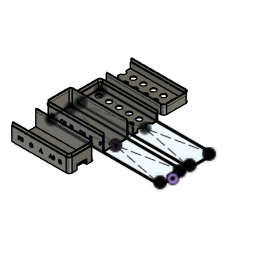
harpcase_v3 (Autodesk Fusion 360 design; units mm, degrees)
Autodesk Fusion 360 part; units mm, degrees
sketch "Sketch1" plane through (0, 0, 0) normal (0, 0, 1) x (1, 0, 0)
  line L0 (167.5, 35) -> (-167.5, 35)
  line L1 (-172.5, 30) -> (-172.5, -30)
  line L2 (-167.5, -35) -> (167.5, -35)
  line L3 (172.5, -30) -> (172.5, 30)
  line L4 (172.5, 35) -> (-172.5, -35) construction
  line L5 (-172.5, 35) -> (172.5, -35) construction
  line L6 (0, 0) -> (0, 91) construction
  line L7 (167.5, 126) -> (-167.5, 126)
  line L8 (-172.5, 121) -> (-172.5, 61)
  line L9 (-167.5, 56) -> (167.5, 56)
  line L10 (172.5, 61) -> (172.5, 121)
  line L11 (172.5, 126) -> (-172.5, 56) construction
  line L12 (-172.5, 126) -> (172.5, 56) construction
  arc A0 (-167.5, 126) -> (-172.5, 121) centre (-167.5, 121) ccw
  arc A1 (172.5, 121) -> (167.5, 126) centre (167.5, 121) ccw
  arc A2 (167.5, 56) -> (172.5, 61) centre (167.5, 61) ccw
  arc A3 (-172.5, 61) -> (-167.5, 56) centre (-167.5, 61) ccw
  arc A4 (-167.5, 35) -> (-172.5, 30) centre (-167.5, 30) ccw
  arc A5 (-172.5, -30) -> (-167.5, -35) centre (-167.5, -30) ccw
  arc A6 (167.5, -35) -> (172.5, -30) centre (167.5, -30) ccw
  arc A7 (172.5, 30) -> (167.5, 35) centre (167.5, 30) ccw
  line L13 (-176.5417, 121) -> (-176.5417, 61)
  arc A8 (-176.5417, 61) -> (-167.5, 51.9583) centre (-167.5, 61) ccw
  line L14 (-167.5, 51.9583) -> (167.5, 51.9583)
  arc A9 (167.5, 51.9583) -> (176.5417, 61) centre (167.5, 61) ccw
  line L15 (176.5417, 61) -> (176.5417, 121)
  arc A10 (176.5417, 121) -> (167.5, 130.0417) centre (167.5, 121) ccw
  line L16 (167.5, 130.0417) -> (-167.5, 130.0417)
  arc A11 (-167.5, 130.0417) -> (-176.5417, 121) centre (-167.5, 121) ccw
  line L17 (-174.5208, 121) -> (-174.5208, 61)
  arc A12 (-174.5208, 61) -> (-167.5, 53.9792) centre (-167.5, 61) ccw
  line L18 (-167.5, 53.9792) -> (167.5, 53.9792)
  arc A13 (167.5, 53.9792) -> (174.5208, 61) centre (167.5, 61) ccw
  line L19 (174.5208, 61) -> (174.5208, 121)
  arc A14 (174.5208, 121) -> (167.5, 128.0208) centre (167.5, 121) ccw
  line L20 (167.5, 128.0208) -> (-167.5, 128.0208)
  arc A15 (-167.5, 128.0208) -> (-174.5208, 121) centre (-167.5, 121) ccw
  line L21 (-176.5417, 30) -> (-176.5417, -30)
  arc A16 (-176.5417, -30) -> (-167.5, -39.0417) centre (-167.5, -30) ccw
  line L22 (-167.5, -39.0417) -> (167.5, -39.0417)
  arc A17 (167.5, -39.0417) -> (176.5417, -30) centre (167.5, -30) ccw
  line L23 (176.5417, -30) -> (176.5417, 30)
  arc A18 (176.5417, 30) -> (167.5, 39.0417) centre (167.5, 30) ccw
  line L24 (167.5, 39.0417) -> (-167.5, 39.0417)
  arc A19 (-167.5, 39.0417) -> (-176.5417, 30) centre (-167.5, 30) ccw
  line L25 (-174.5208, 30) -> (-174.5208, -30)
  arc A20 (-174.5208, -30) -> (-167.5, -37.0208) centre (-167.5, -30) ccw
  line L26 (-167.5, -37.0208) -> (167.5, -37.0208)
  arc A21 (167.5, -37.0208) -> (174.5208, -30) centre (167.5, -30) ccw
  line L27 (174.5208, -30) -> (174.5208, 30)
  arc A22 (174.5208, 30) -> (167.5, 37.0208) centre (167.5, 30) ccw
  line L28 (167.5, 37.0208) -> (-167.5, 37.0208)
  arc A23 (-167.5, 37.0208) -> (-174.5208, 30) centre (-167.5, 30) ccw
  point P0 (0, 91)
  dimension "d5" = 345
  dimension "d6" = 70
  dimension "d7" = 91
  dimension "d8" = 345
  dimension "d9" = 70
  dimension "d11" = 5
  dimension "d12" = 5
  dimension "d14" = 4.0417
  dimension "d15" = 2.0208
  dimension "d16" = 4.0417
  dimension "d17" = 2.0208
  constraint horizontal L0
  constraint perpendicular L0 L1
  constraint parallel L0 L2
  constraint parallel L1 L3
  constraint coincident L4 L6.start
  constraint coincident L5 L6.start
  constraint coincident L6.start origin
  constraint perpendicular L0 L6
  constraint horizontal L7
  constraint perpendicular L7 L8
  constraint parallel L7 L9
  constraint parallel L8 L10
  constraint coincident L11 P0
  constraint coincident L12 P0
  constraint coincident P0 L6.end
  constraint coincident L12.start L8
  constraint coincident L12.start L7
  constraint tangent L8 A0
  constraint tangent L7 A0
  constraint coincident L11.start L7
  constraint coincident L11.start L10
  constraint tangent L7 A1
  constraint tangent L10 A1
  constraint equal A0 A1
  constraint coincident L12.end L9
  constraint coincident L12.end L10
  constraint tangent L9 A2
  constraint tangent L10 A2
  constraint equal A0 A2
  constraint coincident L11.end L9
  constraint coincident L11.end L8
  constraint tangent L9 A3
  constraint tangent L8 A3
  constraint equal A0 A3
  constraint coincident L5.start L1
  constraint coincident L5.start L0
  constraint tangent L1 A4
  constraint tangent L0 A4
  constraint coincident L4.end L2
  constraint coincident L4.end L1
  constraint tangent L2 A5
  constraint tangent L1 A5
  constraint equal A4 A5
  constraint coincident L5.end L2
  constraint coincident L5.end L3
  constraint tangent L2 A6
  constraint tangent L3 A6
  constraint equal A4 A6
  constraint coincident L4.start L0
  constraint coincident L4.start L3
  constraint tangent L0 A7
  constraint tangent L3 A7
  constraint equal A4 A7
  measures "d5" distance of L4.end L5.end
  measures "d6" distance of L5.start L4.end
  measures "d7" distance of L6.start P0
  measures "d8" distance of L11.end L12.end
  measures "d9" distance of L12.start L11.end
  measures "d11" radius of A0
  measures "d12" radius of A4
extrude "Extrude1" add sketch "Sketch1" along normal blind 2.425 contours L0 L1 L2 L3 A4 A5 A6 A7 | L7 L8 L9 L10 A0 A1 A2 A3 makes body 1 at (55.8333, 79.3333, 0) makes body 2 at (55.8333, -11.6667, 0)
extrude "Extrude2" add sketch "Sketch1" along normal blind 50.4 contours L25 A20 L26 A21 L27 A22 L28 A23 bodies 2
extrude "Extrude3" add sketch "Sketch1" along normal blind 42 contours L21 A16 L22 A17 L23 A18 L24 A19 bodies 2
extrude "Extrude4" add sketch "Sketch1" along normal blind 19.6 contours L17 A12 L18 A13 L19 A14 L20 A15 bodies 1
extrude "Extrude5" add sketch "Sketch1" along normal blind 28 contours L13 A8 L14 A9 L15 A10 L16 A11 bodies 1
ref_plane "WorkPlane1" through (176.5417, 0, 21) normal (1, 0, 0) x (0, 1, 0)
sketch "Sketch2" plane through (176.5417, 0, 0) normal (1, 0, 0) x (0, 1, 0)
  line L0 (0, 0) -> (15, 0)
  line L1 (15, 0) -> (15, 15)
  line L2 (15, 15) -> (0, 15)
  line L3 (0, 15) -> (0, 0)
  line L4 (0, 0) -> (-15, 0)
  line L5 (-15, 0) -> (-15, 15)
  line L6 (-15, 15) -> (0, 15)
  line L7 (0, 15) -> (0, 0)
  dimension "d35" = 15
  dimension "d36" = 15
  dimension "d38" = 15
  dimension "d39" = 15
  constraint horizontal L0
  constraint vertical L1
  constraint horizontal L2
  constraint vertical L3
  constraint coincident L0.start L3.end
  constraint horizontal L4
  constraint vertical L5
  constraint horizontal L6
  constraint vertical L7
  measures "d35" distance of L0.start L0.end
  measures "d36" distance of L0.start L2.end
  measures "d38" distance of L0.start L4.end
  measures "d39" distance of L0.start L2.end
extrude "Extrude6" cut sketch "Sketch2" against normal blind 10 bodies 2
ref_plane "WorkPlane2" through (0, 91, 2.425) normal (0, 0, 1) x (1, 0, 0)
sketch "Sketch3" plane through (0, 0, 2.425) normal (0, 0, 1) x (1, 0, 0)
  line L0 (167.5, 126) -> (-167.5, 126)
  line L1 (-172.5, 121) -> (-172.5, 61)
  line L2 (-167.5, 56) -> (172.5, 56)
  line L3 (172.5, 62.1164) -> (172.5, 121)
  line L4 (172.5, 126) -> (-172.5, 56) construction
  line L5 (-172.5, 126) -> (166.5058, 57.2162) construction
  arc A0 (-167.5, 126) -> (-172.5, 121) centre (-167.5, 121) ccw
  arc A1 (-172.5, 61) -> (-167.5, 56) centre (-167.5, 61) ccw
  arc A2 (166.5058, 57.2162) -> (172.5, 62.1164) centre (167.5, 62.1164) ccw
  arc A3 (172.5, 121) -> (167.5, 126) centre (167.5, 121) ccw
  line L6 (0, 126) -> (0, 56) construction
  line L7 (172.5, 91.5582) -> (-172.5, 91) construction
  line L8 (0, 56) -> (-155, 56) construction
  line L9 (-172.5, 91) -> (-172.4741, 75) construction
  line L10 (-155, 56) -> (-155, 77.7) construction
  circle A4 centre (-155, 77.7) radius 8.1
  line L11 (-155, 77.7) -> (-155.043, 104.3) construction
  circle A5 centre (-155.043, 104.3) radius 8.1
  circle A6 centre (-124.043, 104.3) radius 8.1
  circle A7 centre (-124, 77.7) radius 8.1
  circle A8 centre (-93.043, 104.3) radius 8.1
  circle A9 centre (-93, 77.7) radius 8.1
  circle A10 centre (-62.043, 104.3) radius 8.1
  circle A11 centre (-62, 77.7) radius 8.1
  circle A12 centre (-31.043, 104.3) radius 8.1
  circle A13 centre (-31, 77.7) radius 8.1
  circle A14 centre (-0.043, 104.3) radius 8.1
  circle A15 centre (0, 77.7) radius 8.1
  circle A16 centre (30.957, 104.3) radius 8.1
  circle A17 centre (31, 77.7) radius 8.1
  circle A18 centre (61.957, 104.3) radius 8.1
  circle A19 centre (62, 77.7) radius 8.1
  circle A20 centre (92.957, 104.3) radius 8.1
  circle A21 centre (93, 77.7) radius 8.1
  circle A22 centre (123.957, 104.3) radius 8.1
  circle A23 centre (124, 77.7) radius 8.1
  circle A24 centre (154.957, 104.3) radius 8.1
  circle A25 centre (155, 77.7) radius 8.1
  point P0 (0, 91)
  point P1 (0, 91)
  dimension "d43" = 345
  dimension "d44" = 70
  dimension "d45" = 5
  dimension "d46" = 155
  dimension "d47" = 16
  dimension "d48" = 21.7
  dimension "d49" = 16.2
  dimension "d50" = 26.6
  dimension "d51" = 16.2
  dimension "d54" = 310
  dimension "d55" = 0
  constraint horizontal L0
  constraint perpendicular L0 L1
  constraint parallel L0 L2
  constraint parallel L1 L3
  constraint coincident L4 P1
  constraint coincident L5 P1
  constraint coincident L5.start L0
  constraint coincident L5.start L1
  constraint tangent L0 A0
  constraint tangent L1 A0
  constraint coincident L4.end L1
  constraint coincident L4.end L2
  constraint tangent L1 A1
  constraint tangent L2 A1
  constraint equal A0 A1
  constraint coincident L2.end L3
  constraint coincident L2.end L5
  constraint tangent L3 A2
  constraint tangent L5 A2
  constraint equal A0 A2
  constraint coincident L4.start L3
  constraint coincident L4.start L0
  constraint tangent L3 A3
  constraint tangent L0 A3
  constraint equal A0 A3
  constraint coincident P1 P0
  constraint midpoint L0 L6.start
  constraint coincident L2 L6.end
  constraint perpendicular L2 L6
  constraint midpoint L3 L7.start
  constraint midpoint L1 L7.end
  constraint perpendicular L6 L8
  constraint perpendicular L7 L9
  constraint perpendicular L8 L10
  constraint coincident L10.end A4.centre
  constraint perpendicular L7 L11
  constraint coincident L11.end A5.centre
  measures "d43" distance of L4.end L2.end
  measures "d44" distance of L5.start L4.end
  measures "d45" radius of A0
  measures "d46" distance of L6.end L8.end
  measures "d47" distance of L7.end L9.end
  measures "d48" distance of L8.end L10.end
  measures "d49" diameter of A4
  measures "d50" distance of L10.end L11.end
  measures "d51" diameter of A5
extrude "Extrude7" cut sketch "Sketch3" against normal blind 10 bodies 1
ref_plane "WorkPlane3" through (0, -39.0417, 21) normal (0, -1, 0) x (1, 0, 0)
sketch "Sketch4" plane through (0, -39.0417, 0) normal (0, -1, 0) x (-1, 0, 0)
  line L0 (160, -10) -> (150, -10) construction
  line L1 (150, -10) -> (150, -25) construction
  line L2 (150, -25) -> (160, -25) construction
  line L3 (160, -25) -> (160, -10) construction
  line L4 (130, -10) -> (120, -10) construction
  line L5 (120, -10) -> (120, -25) construction
  line L6 (120, -25) -> (130, -25) construction
  line L7 (130, -25) -> (130, -10) construction
  line L8 (100, -10) -> (90, -10) construction
  line L9 (90, -10) -> (90, -25) construction
  line L10 (90, -25) -> (100, -25) construction
  line L11 (100, -25) -> (100, -10) construction
  line L12 (70, -10) -> (60, -10) construction
  line L13 (60, -10) -> (60, -25) construction
  line L14 (60, -25) -> (70, -25) construction
  line L15 (70, -25) -> (70, -10) construction
  line L16 (40, -10) -> (30, -10) construction
  line L17 (30, -10) -> (30, -25) construction
  line L18 (30, -25) -> (40, -25) construction
  line L19 (40, -25) -> (40, -10) construction
  line L20 (10, -10) -> (0, -10) construction
  line L21 (0, -10) -> (0, -25) construction
  line L22 (0, -25) -> (10, -25) construction
  line L23 (10, -25) -> (10, -10) construction
  line L24 (-20, -10) -> (-30, -10) construction
  line L25 (-30, -10) -> (-30, -25) construction
  line L26 (-30, -25) -> (-20, -25) construction
  line L27 (-20, -25) -> (-20, -10) construction
  line L28 (-55, -10) -> (-65, -10) construction
  line L29 (-65, -10) -> (-65, -25) construction
  line L30 (-65, -25) -> (-55, -25) construction
  line L31 (-55, -25) -> (-55, -10) construction
  line L32 (-85, -10) -> (-95, -10) construction
  line L33 (-95, -10) -> (-95, -25) construction
  line L34 (-95, -25) -> (-85, -25) construction
  line L35 (-85, -25) -> (-85, -10) construction
  line L36 (-115, -10) -> (-125, -10) construction
  line L37 (-125, -10) -> (-125, -25) construction
  line L38 (-125, -25) -> (-115, -25) construction
  line L39 (-115, -25) -> (-115, -10) construction
  line L40 (-145, -10) -> (-155, -10) construction
  line L41 (-155, -10) -> (-155, -25) construction
  line L42 (-155, -25) -> (-145, -25) construction
  line L43 (-145, -25) -> (-145, -10) construction
  dimension "d60" = 10
  dimension "d61" = 10
  dimension "d62" = 10
  dimension "d63" = 10
  dimension "d64" = 10
  dimension "d65" = 10
  dimension "d66" = 10
  dimension "d67" = 10
  dimension "d68" = 10
  dimension "d69" = 10
  dimension "d70" = 10
  text T0 "C" font "Arial" height 10 align left top in box 10 x 15 at (160, -10) x (-1, 0) y (0, -1) spacing 1 kerned
  text T1 "C#" font "Arial" height 10 align left top in box 10 x 15 at (130, -10) x (-1, 0) y (0, -1) spacing 1 kerned
  text T2 "D" font "Arial" height 10 align left top in box 10 x 15 at (100, -10) x (-1, 0) y (0, -1) spacing 1 kerned
  text T3 "D#" font "Arial" height 10 align left top in box 10 x 15 at (70, -10) x (-1, 0) y (0, -1) spacing 1 kerned
  text T4 "E" font "Arial" height 10 align left top in box 10 x 15 at (40, -10) x (-1, 0) y (0, -1) spacing 1 kerned
  text T5 "F\n" font "Arial" height 10 align left top in box 10 x 15 at (10, -10) x (-1, 0) y (0, -1) spacing 1 kerned
  text T6 "F#" font "Arial" height 10 align left top in box 10 x 15 at (-20, -10) x (-1, 0) y (0, -1) spacing 1 kerned
  text T7 "G" font "Arial" height 10 align left top in box 10 x 15 at (-55, -10) x (-1, 0) y (0, -1) spacing 1 kerned
  text T8 "A" font "Arial" height 10 align left top in box 10 x 15 at (-85, -10) x (-1, 0) y (0, -1) spacing 1 kerned
  text T9 "A#" font "Arial" height 10 align left top in box 10 x 15 at (-115, -10) x (-1, 0) y (0, -1) spacing 1 kerned
  text T10 "B" font "Arial" height 10 align left top in box 10 x 15 at (-145, -10) x (-1, 0) y (0, -1) spacing 1 kerned
extrude "Extrude8" cut sketch "Sketch4" against normal blind 1.5 text T0 T1 T2 T3 T4 T5 T6 T7 T8 T9 T10 bodies 2
split "Split1" by plane through (0, 0, 0) normal (1, 0, 0) bodies 2 makes body 3 at (55.5139, -5, 0)
split "Split2" by plane through (0, 0, 0) normal (1, 0, 0) bodies 1 makes body 4 at (86.6172, 124.1535, 0)
move_body "Move1" bodies 3 to x (1, 0, 0) y (0, 1, 0) z (0, 0, 1) at (-170, -110, 0)
move_body "Move2" bodies 4 to x (1, 0, 0) y (0, 1, 0) z (0, 0, 1) at (-180, 100, 0)
move_face "OffsetFaces1" offset -0.2 10 faces at (-55.8333, 128.0208, 22.4) (-174.5208, 101, 22.4) (-170.7171, 54.7596, 25.2) (-111.6667, 53.9792, 22.4) (-170.1094, 127.5179, 25.2) (-68.3333, 228.0208, 22.4) (-5.4792, 181, 22.4) (-5.4871, 221.3341, 22.4) (-6.2596, 157.7829, 25.2) (-124.1667, 153.9792, 22.4) on bodies 1 4
equation "harpL = 345 mm"
equation "harpW = 70 mm"
equation "harpH = 70 mm"
equation "gap = harpH * 1.30"
equation "d5 = harpL"
equation "d6 = harpW"
equation "d7 = gap"
equation "d8 = harpL"
equation "d9 = harpW"
equation "harpR = 5 mm"
equation "d11 = harpR"
equation "d12 = harpR"
equation "harpT = ( harpH + harpW + harpL ) / 3 * 0.025"
equation "d14 = harpT"
equation "d15 = harpT / 2"
equation "d16 = harpT"
equation "d17 = harpT / 2"
equation "seempercent = 0.6"
equation "baseH = harpH * seempercent"
equation "capH = harpH * ( 1 - seempercent )"
equation "olp = 0.3"
equation "overlapH = capH * olp"
equation "d23 = harpT * 0.6"
equation "d25 = baseH + overlapH"
equation "d27 = baseH"
equation "d29 = capH - overlapH"
equation "d31 = capH"
equation "cutgap = 10 mm"
equation "d35 = cutSL"
equation "d36 = cutSL"
equation "cutSL = 15 mm"
equation "d38 = cutSL"
equation "d39 = cutSL"
equation "d43 = harpL"
equation "d44 = harpW"
equation "d45 = harpR"
equation "d48 = 22 mm - 0.3 mm"
